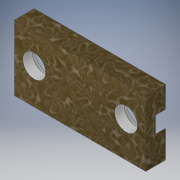
# Autodesk Inventor part: reverse gear bearing keeper
Saved by Autodesk Inventor 2017 (Build 210142000, 142)
## iProperties
Created: 2018-10-30
Part Number: reverse gear bearing keeper
Material: Generic
Document SubType Name: Modeling
Designer: User
Density: 1 g/cm^3
Appearance: Default
Author: User
Autodesk Inventor part; units mm, degrees
ref_plane "YZ Plane" through (0, 0, 0) normal (1, 0, 0) x (0, 1, 0)
ref_plane "XZ Plane" through (0, 0, 0) normal (0, 1, 0) x (-1, 0, 0)
ref_plane "XY Plane" through (0, 0, 0) normal (0, 0, 1) x (1, 0, 0)
sketch "Sketch1" plane through (0, 0, 0) normal (0, 1, 0) x (-1, 0, 0)
  line L0 (0, 0) -> (0, -10)
  line L1 (0, -10) -> (-20, -10)
  line L2 (-20, -10) -> (-20, 0)
  line L3 (-20, 0) -> (0, 0)
  arc A0 (0, -3.3117) -> (0, -5.8117) centre (-3, -4.5617) ccw
  arc A1 (-20, -5.8117) -> (-20, -3.3117) centre (-17, -4.5617) ccw
  line L4 (-10, 0) -> (-10, -10) construction
  circle A2 centre (-3, -4.5617) radius 1.75
  circle A3 centre (-17, -4.5617) radius 1.75
  dimension "d2" = 10
  dimension "d3" = 20
  dimension "d5" = 6.5
  dimension "d8" = 7
  dimension "d9" = 7
  dimension "d11" = 3.5
  dimension "d12" = 3.5
  dimension "d13" = 10
  dimension "d14" = 3.3117
  dimension "d15" = 4.5617
  constraints: 10 end point, 4 centre point, 4 point on circle, 4 point on line, 2 coincident, 2 midpoint, 2 perpendicular, 1 equal radius, 1 parallel, 1 vertical
  measures "d2" distance of L1.end L2.end
  measures "d3" distance of L2.end L0.start
  measures "d5" diameter of A1
  measures "d8" distance from line of L4 A0.centre
  measures "d9" distance from line of L4 A1.centre
  measures "d11" diameter of A2
  measures "d12" diameter of A3
  measures "d13" distance between parallel lines of L0 L4
  measures "d14" distance from line of A0.start L3
  measures "d15" distance from line of A1.centre L3
extrude "Extrusion1" add sketch "Sketch1" along normal blind 1.5 contours L0 A0 | A1 L2
extrude "Extrusion2" add sketch "Sketch1" along normal blind 3 contours L0 A0 L1 L2 A1 L3
body "Solid1"
